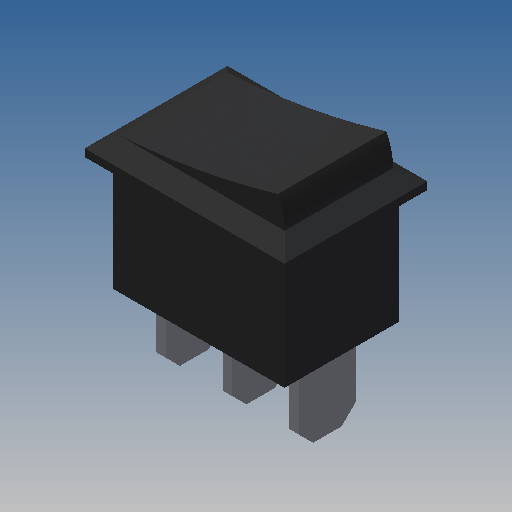
# Autodesk Inventor part: Toggle switch
Saved by Autodesk Inventor 2017 (Build 210142000, 142)
## iProperties
Created: 2016-10-18
Part Number: Toggle switch
Material: Generic
Document SubType Name: Modeling
Designer: James Yelland
Density: 1 g/cm^3
Appearance: Default
Author: James Yelland
Autodesk Inventor part; units mm, degrees
ref_plane "YZ Plane" through (0, 0, 0) normal (1, 0, 0) x (0, 1, 0)
ref_plane "XZ Plane" through (0, 0, 0) normal (0, 1, 0) x (-1, 0, 0)
ref_plane "XY Plane" through (0, 0, 0) normal (0, 0, 1) x (1, 0, 0)
sketch "Sketch1" plane through (0, 0, 0) normal (0, 1, 0) x (-1, 0, 0)
  line L0 (-9, 6) -> (-9, -6)
  line L1 (-9, -6) -> (9, -6)
  line L2 (9, -6) -> (9, 6)
  line L3 (9, 6) -> (-9, 6)
  line L4 (-9, 6) -> (9, -6) construction
  line L5 (-9, -6) -> (9, 6) construction
  point P0 (0, 0)
  dimension "d0" = 12
  dimension "d1" = 18
  constraints: 12 end point, 2 midpoint, 2 parallel, 1 perpendicular, 1 vertical
  measures "d0" distance of L0.start L0.end
  measures "d1" distance of L1.end L0.end
extrude "Extrusion1" add sketch "Sketch1" along normal blind 12
sketch "Sketch2" plane through (0, 12, 0) normal (0, 1, 0) x (1, 0, 0)
  line L0 (10.5, -7.5) -> (10.5, 7.5)
  line L1 (10.5, 7.5) -> (-10.5, 7.5)
  line L2 (-10.5, 7.5) -> (-10.5, -7.5)
  line L3 (-10.5, -7.5) -> (10.5, -7.5)
  line L4 (10.5, -7.5) -> (-10.5, 7.5) construction
  line L5 (10.5, 7.5) -> (-10.5, -7.5) construction
  point P0 (0, 0)
  dimension "d4" = 15
  dimension "d5" = 21
  constraints: 12 end point, 2 midpoint, 2 parallel, 1 perpendicular, 1 vertical
  measures "d4" distance of L0.start L0.end
  measures "d5" distance of L1.end L0.end
extrude "Extrusion2" add sketch "Sketch2" along normal blind 2
chamfer "Chamfer1" distance 1.8 distance2 1.2 1 edges at (10.5, 14, 0) measured on face at (-3.5, 14, -2.5)
chamfer "Chamfer2" distance 1.8 distance2 1.2 1 edges at (-0.9, 14, 7.5) measured on face at (-4.1, 14, -2.5)
chamfer "Chamfer3" distance 1.8 distance2 1.2 1 edges at (-10.5, 14, -0.9) measured on face at (-4.1, 14, -3.1)
chamfer "Chamfer4" distance 1.8 distance2 1.2 1 edges at (0, 14, -7.5) measured on face at (2.9, 14, 1.3)
sketch "Sketch3" plane through (0, 14, 0) normal (0, 1, 0) x (1, 0, 0)
  line L0 (-8.7, 5.7) -> (8.7, 5.7) projected
  line L1 (-8.7, -5.7) -> (-8.7, 5.7) projected
  line L2 (8.7, -5.7) -> (-8.7, -5.7) projected
  line L3 (8.7, 5.7) -> (8.7, -5.7) projected
  point P0 (0, 0)
extrude "Extrusion3" add sketch "Sketch3" along normal blind 3
sketch "Sketch4" plane through (-8.7, 14, 5.7) normal (0, 0, 1) x (1, 0, 0)
  line L0 (17.4, 0) -> (0, 0) projected
  line L1 (17.4, 0) -> (17.4, 3) projected
  line L2 (0, 3) -> (17.4, 3) projected
  line L3 (0, 0) -> (0, 3) projected
  line L4 (17.4, 0) -> (17.4, 3)
  line L5 (17.4, 3) -> (0, 3)
  line L6 (0, 3) -> (0, 0)
  line L7 (0, 0) -> (17.4, 0)
  line L8 (17.4, 0) -> (16.7, 0)
  line L9 (17.4, 0) -> (0, 0) projected
  line L10 (16.7, 0) -> (16.7, 3)
  line L11 (0, 3) -> (17.4, 3) projected
  arc A0 (0, 0) -> (16.7, 3) centre (-4.649, 73.861) ccw
  arc A1 (17.4, 0) -> (16.7, 3) centre (10.8425, 0.0516) ccw
  point P0 (8.7, -14)
  dimension "d24" = 0.7
  constraints: 12 end point, 4 point on circle, 3 collinear, 2 centre point, 2 point on line, 1 perpendicular, 1 vertical
  measures "d24" distance of L7.end L8.end
extrude "Extrusion4" cut sketch "Sketch4" against normal through all contours A1 L2 L1 | A0 L3 L2
sketch "Sketch5" plane through (0, 0, 0) normal (0, -1, 0) x (1, 0, 0)
  line L0 (0.5, -3) -> (0.5, 3)
  line L1 (0.5, 3) -> (-0.5, 3)
  line L2 (-0.5, 3) -> (-0.5, -3)
  line L3 (-0.5, -3) -> (0.5, -3)
  line L4 (0.5, -3) -> (-0.5, 3) construction
  line L5 (0.5, 3) -> (-0.5, -3) construction
  line L6 (0, 0) -> (-7, 0)
  line L7 (0, 0) -> (7, 0)
  line L8 (-6.5, -3) -> (-6.5, 3)
  line L9 (-6.5, 3) -> (-7.5, 3)
  line L10 (-7.5, 3) -> (-7.5, -3)
  line L11 (-7.5, -3) -> (-6.5, -3)
  line L12 (-6.5, -3) -> (-7.5, 3) construction
  line L13 (-6.5, 3) -> (-7.5, -3) construction
  line L14 (7.5, -3) -> (7.5, 3)
  line L15 (7.5, 3) -> (6.5, 3)
  line L16 (6.5, 3) -> (6.5, -3)
  line L17 (6.5, -3) -> (7.5, -3)
  line L18 (7.5, -3) -> (6.5, 3) construction
  line L19 (7.5, 3) -> (6.5, -3) construction
  dimension "d27" = 6
  dimension "d28" = 1
  dimension "d29" = 7
  dimension "d30" = 7
  dimension "d31" = 1
  dimension "d32" = 1
  dimension "d41" = 6
  dimension "d42" = 6
  constraints: 40 end point, 6 midpoint, 6 parallel, 5 perpendicular, 2 vertical, 1 horizontal
  measures "d27" distance of L0.start L0.end
  measures "d28" distance of L1.end L0.end
  measures "d29" distance of L6.start L6.end
  measures "d30" distance of L6.start L7.end
  measures "d31" distance of L9.end L8.end
  measures "d32" distance of L15.end L14.end
  measures "d41" distance of L15.end L16.end
  measures "d42" distance of L8.start L8.end
extrude "Extrusion5" add sketch "Sketch5" along normal blind 8
chamfer "Chamfer5" distance 1.5 angle 45 6 edges at (7, -8, -3) (7, -8, 3) (0, -8, 3) (-7, -8, 3) (-7, -8, -3) (0, -8, -3)
body "Solid1"
